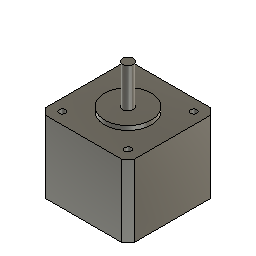
0616e7d9-f380-47b4-a429-0148fa68df5b (Autodesk Fusion 360 design; units mm, degrees)
Autodesk Fusion 360 part; units mm, degrees
sketch "Sketch1" plane through (0, 0, 0) normal (0, 0, 1) x (1, 0, 0)
  line L0 (21, 21) -> (-21, 21)
  line L1 (-21, 21) -> (-21, -21)
  line L2 (-21, -21) -> (21, -21)
  line L3 (21, -21) -> (21, 21)
  line L4 (21, 21) -> (-21, -21) construction
  line L5 (-21, 21) -> (21, -21) construction
  circle A0 centre (0, 0) radius 11
  circle A1 centre (0, 0) radius 2.5
  circle A2 centre (-15.5, 15.5) radius 1.5
  circle A3 centre (15.5, 15.5) radius 1.5
  circle A4 centre (15.5, -15.5) radius 1.5
  circle A5 centre (-15.5, -15.5) radius 1.5
  line L6 (-15.5, -15.5) -> (-15.5, 15.5) construction
  line L7 (15.5, 15.5) -> (-15.5, 15.5) construction
  line L8 (15.5, -15.5) -> (15.5, 15.5) construction
  line L9 (-15.5, -15.5) -> (15.5, -15.5) construction
  dimension "d1" = 42
  dimension "d2" = 42
  dimension "d3" = 22
  dimension "d4" = 5
  dimension "d12" = 3
  dimension "d13" = 3
  dimension "d14" = 3
  dimension "d15" = 3
  dimension "d16" = 31
  constraint horizontal L0
  constraint perpendicular L0 L1
  constraint parallel L0 L2
  constraint parallel L1 L3
  constraint coincident L4 A0.centre
  constraint coincident L5 A0.centre
  constraint coincident A0.centre A1.centre
  constraint coincident L5 A2.centre
  constraint coincident L4 A3.centre
  constraint coincident L5 A4.centre
  constraint coincident L4 A5.centre
  constraint coincident A5.centre L6.start
  constraint coincident A2.centre L6.end
  constraint coincident A3.centre L7.start
  constraint coincident A4.centre L8.start
  constraint vertical L6
  constraint horizontal L7
  constraint vertical L8
  measures "d1" distance of L1.end L2.end
  measures "d2" distance of L0.end L1.end
  measures "d3" diameter of A0
  measures "d4" diameter of A1
  measures "d12" diameter of A2
  measures "d13" diameter of A3
  measures "d14" diameter of A4
  measures "d15" diameter of A5
  measures "d16" vertical distance of A2.centre A5.centre
extrude "Extrude1" add sketch "Sketch1" against normal blind 34 contours L0 L1 L2 L3 | A0 | A1
extrude "Extrude2" add sketch "Sketch1" along normal blind 2 contours A0
extrude "Extrude3" add sketch "Sketch1" along normal blind 20.5 contours A1
chamfer "Chamfer1" distance 3 angle 45 4 edges at (21, -21, -17) (-21, -21, -17) (-21, 21, -17) (21, 21, -17)
